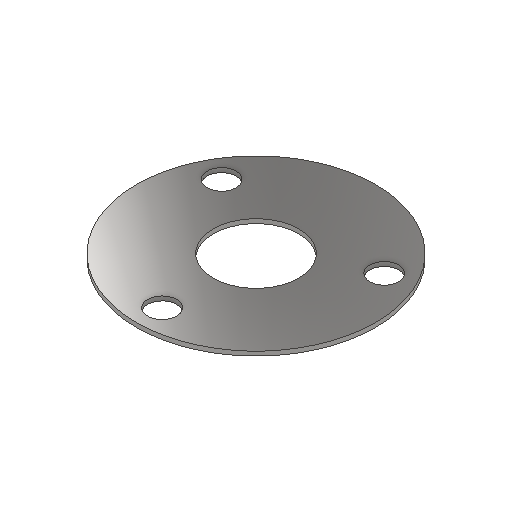
# Autodesk Inventor part: B_holder_up_5
Saved by Autodesk Inventor 2026.2 (Build 302298000, 298)
## iProperties
Created: 2026-02-20
Part Number: B_holder_up_5
Material: ステンレス鋼 440C
Document SubType Name: Modeling
Designer: zetsu
Density: 7.75 g/cm^3
Appearance: 半つや出し
Author: zetsu
Autodesk Inventor part; units mm, degrees
ref_plane "YZ Plane" through (0, 0, 0) normal (1, 0, 0) x (0, 1, 0)
ref_plane "XZ Plane" through (0, 0, 0) normal (0, 1, 0) x (-1, 0, 0)
ref_plane "XY Plane" through (0, 0, 0) normal (0, 0, 1) x (1, 0, 0)
sketch "スケッチ1" plane through (0, 0, 0) normal (0, 1, 0) x (-1, 0, 0)
  circle A0 centre (0, 0) radius 14
  dimension "d0" = 28
  constraints: 1 centre point, 1 coincident
  measures "d0" diameter of A0
extrude "押し出し1" add sketch "スケッチ1" along normal blind 0.5
sketch "スケッチ2" plane through (0, 0.5, 0) normal (0, 1, 0) x (1, 0, 0)
  circle A0 centre (0, -11) radius 1.7
  circle A1 centre (9.5263, 5.5) radius 1.7
  circle A2 centre (-9.5263, 5.5) radius 1.7
  point P0 (0, 0)
  dimension "d4" = 3.4
  dimension "d12" = 11
  dimension "d15" = 360
  constraints: 3 centre point, 7 other
  measures "d4" diameter of A0
  measures "d12" distance of A0.centre point (0, 0)
extrude "押し出し2" cut sketch "スケッチ2" against normal through all
sketch "スケッチ3" plane through (0, 0.5, 0) normal (0, 1, 0) x (1, 0, 0)
  circle A0 centre (0, 0) radius 5
  dimension "d9" = 10
  constraints: 1 centre point, 1 coincident
  measures "d9" diameter of A0
extrude "押し出し3" cut sketch "スケッチ3" against normal through all
